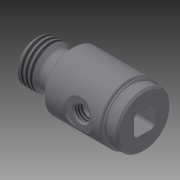
# Autodesk Inventor part: 02R0101_NR_rod_guide
Saved by Autodesk Inventor 2013 (Build 170138000, 138)
## iProperties
Category: PARTsolutions
Company: BIMBA
Created: 2013-01-26
Part Number: 02R0101_NR_rod_guide
Material: Generic
Catalog Web Link: www.cadenas.de
Description: NR Rod Guide-Original Line Cylinders
Vendor: BIMBA
Document SubType Name: Modeling
Designer: actoennies
Manufacturer: BIMBA
Density: 1 g/cm^3
Mass: 3.51503 g
Surface Area: 23.3028 cm^2
Volume: 3.51503 cm^3
PSOL_IDENT_0: {\\10.0.0.242\data_v9\23d-libs\bimba\bimba\bimba_imperial\bimba_full_line\original_line_cylinders\no
PSOL_IDENT_1: n_rotating_air_cylinders\non_rot_rod_guide.prj},201 {VTYP=3D},{NB=02R0101_NR_rod_guide},{LINA=02R010
PSOL_IDENT_2: 1_NR_rod_guide},{NN=NR Rod Guide},{DATE=20.08.2011 07:16:43},{GEOMDATE=16.08.2011 05:39:00},{VERSION
PSOL_IDENT_3: =},{LINEID=30},{LINESUBID=-1},{WBVAR=MNT,DXDE,K,MB}  {NB=02R0101_NR_rod_guide},{LINA=02R0101_NR_rod_
PSOL_IDENT_4: guide},{KT=DUMMY},{PN=02R0101},{BORE=0.56250000},{BOREPN=02},{MNT=},{MNTALG='' , 'Front Nose'},{ACTI
PSOL_IDENT_5: NG=R},{ACTINGALG=R},{DXDE=1},{NR=},{NRALG= '' , 'N/A' },{K=},{T1=},{T2=},{T3=},{T4=},{MB=1},{A1=1.15
PSOL_IDENT_6: 60},{A1N=1.0310},{A1P=1.1560},{A1B=0.0000},{A2=0.3750},{A2N=0.3750},{A2P=0.3750},{A3=0.6250},{A3N=0.
PSOL_IDENT_7: 1250},{A3P=0.6250},{A4=0.1570},{A4N=0.5310},{A4P=0.1570},{A5=0.0250},{A6=0.0000},{A6N=0.2810},{A6P=0
PSOL_IDENT_8: .0000},{A7=0.5000},{A7N=0.6560},{A7P=0.5000},{A8=0.0200},{A8N=0.0200},{A8NR=0.0200},{D1=0.6150},{D1N
PSOL_IDENT_9: =0.6150},{D1P=0.6150},{D1B=0.0000},{D2=0.5725},{D3=0.0000},{D3N=0.4000},{D3P=0.0000},{D4=0.3440},{D4
PSOL_IDENT_10: N=0.2220},{D4P=0.3440},{D4NR=0.3440},{D5=0.1900},{D5N=0.1900},{D5NR=0.1900},{C1=0.030},{C2=0.0200},{
PSOL_IDENT_11: C2N=0.0300},{C2P=0.0200},{C3=0.0100},{C3N=0.0100},{C3P=0.0100},{C4=0.0300},{C4N=0.0300},{C4P=0.0300}
PSOL_IDENT_12: ,{NDM=0.4375},{NDMN=0.4375},{NDMP=0.4375},{TAB=UNF},{D6=0.4355},{D6N=0.4355},{D6P=0.4355},{A9=0.0620
PSOL_IDENT_13: },{A9N=0.0620},{A9P=0.0620},{D7=0.3600},{D7N=0.3600},{D7P=0.3600},{A10=0.0775},{A10N=0.0775},{A10P=0
PSOL_IDENT_14: .0775},{R1=0.0315},{R1N=0.0315},{R1P=0.0315},{D8=0.0000},{D9=0.0000},{D10=0.0000},{A11=0.0000},{A12=
PSOL_IDENT_15: 0.0000},{A13=0.0000},{A14=0.4060},{A14N=0.4060},{A14B=0.0000},{D11=0.0000},{D11N=0.0000},{NDM2=0.190
PSOL_IDENT_16: 0},{NDM2N=0.1900},{NDM2DP=0.0000},{THREAD=0},{HEX=0.2200},{HEXN=0.2200},{S1=0.0000},{B1=0.0000},{B2=
PSOL_IDENT_17: 0.0000},{B22=0.0000},{DB=0.0000},{B3=0.0000},{B4=0.0000},{X1=0.0000},{X2=0.0000},{NDM3=0.0000},{NDM4
PSOL_IDENT_18: =0.0000},{NDM4DP=0.0000},{DD=0.0000},{CB=0.0000},{CBDP=0.0000},{PORT=1},{XT=0.0000},{XT1=0.0000},{XT
PSOL_IDENT_19: 2=0.0000},{NDMH=0.0000},{OD=0.6150},{ID=0.5725},{G=0.0000},{PNUT=0.3750},{TRIM=0},{C11=0.0000},{C22=
PSOL_IDENT_20: 0.0000},{C33=0.0000},{C44=0.0000},{C55=0.0000},{CD1=0.0000},{CD2=0.0000},{CD3=0.0000},{CNDM3=0.0000}
PSOL_IDENT_21: ,{CTAB3=0.0000},{CUSH=0},{XDEDIA=0.19000000},{COR=0.04000000}
CNS_NT: Original Line Cylinders
CNS_NB: 02R0101_NR_rod_guide
CNS_NBSYN: $PN._NR_rod_guide
CNS_LINA: 02R0101_NR_rod_guide
CNS_PN: 02R0101
CNS_BORE: 0.56250000
CNS_BOREPN: 02
CNS_MNT: Front Nose
CNS_MNTALG: '' , 'Front Nose'
CNS_ACTING: R
CNS_ACTINGALG: R
CNS_DXDE: 1
CNS_NRALG: '' , 'N/A'
CNS_K: Standard
CNS_MB: 1
CNS_A1: 1.1560
CNS_A1N: 1.0310
CNS_A1P: 1.1560
CNS_A1B: 0.0000
CNS_A2: 0.3750
CNS_A2N: 0.3750
CNS_A2P: 0.3750
CNS_A3: 0.6250
CNS_A3N: 0.1250
CNS_A3P: 0.6250
CNS_A4: 0.1570
CNS_A4N: 0.5310
CNS_A4P: 0.1570
CNS_A5: 0.0250
CNS_A6: 0.0000
CNS_A6N: 0.2810
CNS_A6P: 0.0000
CNS_A7: 0.5000
CNS_A7N: 0.6560
CNS_A7P: 0.5000
CNS_A8: 0.0200
CNS_A8N: 0.0200
CNS_A8NR: 0.0200
CNS_D1: 0.6150
CNS_D1N: 0.6150
CNS_D1P: 0.6150
CNS_D1B: 0.0000
CNS_D2: 0.5725
CNS_D3: 0.0000
CNS_D3N: 0.4000
CNS_D3P: 0.0000
CNS_D4: 0.3440
CNS_D4N: 0.2220
CNS_D4P: 0.3440
CNS_D4NR: 0.3440
CNS_D5: 0.1900
CNS_D5N: 0.1900
CNS_D5NR: 0.1900
CNS_C1: 0.030
CNS_C2: 0.0200
CNS_C2N: 0.0300
CNS_C2P: 0.0200
CNS_C3: 0.0100
CNS_C3N: 0.0100
CNS_C3P: 0.0100
CNS_C4: 0.0300
CNS_C4N: 0.0300
CNS_C4P: 0.0300
CNS_NDM: 0.4375
CNS_NDMN: 0.4375
CNS_NDMP: 0.4375
CNS_TAB: UNF
CNS_D6: 0.4355
CNS_D6N: 0.4355
CNS_D6P: 0.4355
CNS_A9: 0.0620
CNS_A9N: 0.0620
CNS_A9P: 0.0620
CNS_D7: 0.3600
CNS_D7N: 0.3600
CNS_D7P: 0.3600
CNS_A10: 0.0775
CNS_A10N: 0.0775
CNS_A10P: 0.0775
CNS_R1: 0.0315
CNS_R1N: 0.0315
CNS_R1P: 0.0315
CNS_D8: 0.0000
CNS_D9: 0.0000
CNS_D10: 0.0000
CNS_A11: 0.0000
CNS_A12: 0.0000
CNS_A13: 0.0000
CNS_A14: 0.4060
CNS_A14N: 0.4060
CNS_A14B: 0.0000
CNS_D11: 0.0000
CNS_D11N: 0.0000
CNS_NDM2: 0.1900
CNS_NDM2N: 0.1900
CNS_NDM2DP: 0.0000
CNS_THREAD: 0
CNS_HEX: 0.2200
CNS_HEXN: 0.2200
CNS_S1: 0.0000
CNS_B1: 0.0000
CNS_B2: 0.0000
CNS_B22: 0.0000
CNS_DB: 0.0000
CNS_B3: 0.0000
CNS_B4: 0.0000
CNS_X1: 0.0000
CNS_X2: 0.0000
CNS_NDM3: 0.0000
CNS_NDM4: 0.0000
CNS_NDM4DP: 0.0000
CNS_DD: 0.0000
CNS_CB: 0.0000
CNS_CBDP: 0.0000
CNS_PORT: 1
CNS_XT: 0.0000
CNS_XT1: 0.0000
CNS_XT2: 0.0000
CNS_NDMH: 0.0000
CNS_OD: 0.6150
CNS_ID: 0.5725
CNS_G: 0.0000
CNS_PNUT: 0.3750
CNS_TRIM: 0
CNS_C11: 0.0000
CNS_C22: 0.0000
CNS_C33: 0.0000
CNS_C44: 0.0000
CNS_C55: 0.0000
CNS_CD1: 0.0000
CNS_CD2: 0.0000
CNS_CD3: 0.0000
CNS_CNDM3: 0.0000
CNS_CTAB3: 0.0000
CNS_CUSH: 0.000
CNS_XDEDIA: 0.19000000
CNS_COR: 0.04000000
SUPPLIER: BIMBA
ARTICLENO: 02R0101_NR_rod_guide
BOMINFO: 02R0101_NR_rod_guide
CREATOR: CADENAS GmbH
Title: 02R0101_NR_rod_guide
Author: Cadenas PARTsolutions
Comments: Original Line Cylinders
Autodesk Inventor part; units mm, degrees
sketch "Sketch_2" plane through (0, 0, 0) normal (0, 0, 1) x (1, 0, 0)
  line L0 (9.525, 0) -> (0, 0)
  line L1 (0, 0) -> (0, 4.8006)
  line L2 (0, 4.8006) -> (0.7557, 5.5563)
  line L3 (0.7557, 5.5563) -> (4.6603, 5.5563)
  line L4 (4.6603, 5.5563) -> (5.4159, 4.8006)
  line L5 (5.4159, 4.8006) -> (5.4788, 4.7498)
  arc A0 (5.4788, 4.7498) -> (5.9817, 4.572) centre (5.9817, 5.3721) ccw
  line L6 (5.9817, 4.572) -> (7.1501, 4.572)
  arc A1 (7.1501, 4.572) -> (7.9502, 5.3721) centre (7.1501, 5.3721) ccw
  line L7 (7.9502, 5.3721) -> (7.9502, 5.5309)
  line L8 (7.9502, 5.5309) -> (9.525, 5.5309)
  line L9 (9.525, 5.5309) -> (9.525, 0)
  line L10 (9.525, 0) -> (0, 0)
  constraints: 22 end point, 4 point on circle, 2 centre point
revolve "Revolution1" add sketch "Sketch_2" angle 360 about axis through (9.525, 0, 0) along (1, 0, 0)
thread "Thread1" size "7/16-20 UNF" class "2A" standard "ANSI Unified Screw Threads" full length
sketch "Sketch_3" plane through (0, 0, 0) normal (0, 0, 1) x (1, 0, 0)
  line L0 (29.3624, 0) -> (9.525, 0)
  line L1 (9.525, 0) -> (9.525, 7.0485)
  line L2 (9.525, 7.0485) -> (10.287, 7.8105)
  line L3 (10.287, 7.8105) -> (25.1206, 7.8105)
  line L4 (25.1206, 7.8105) -> (25.3746, 7.5565)
  line L5 (25.3746, 7.5565) -> (25.3746, 6.6357)
  line L6 (25.3746, 6.6357) -> (26.0096, 6.6357)
  line L7 (26.0096, 6.6357) -> (26.6446, 7.2708)
  line L8 (26.6446, 7.2708) -> (28.8544, 7.2708)
  line L9 (28.8544, 7.2708) -> (29.3624, 6.7627)
  line L10 (29.3624, 6.7627) -> (29.3624, 0)
  line L11 (29.3624, 0) -> (9.525, 0)
  constraints: 24 end point
revolve "Revolution2" add sketch "Sketch_3" angle 360 about axis through (29.3624, 0, 0) along (1, 0, 0)
sketch "Sketch_12" plane through (0, 0, 0) normal (0, 1, 0) x (-1, 0, 0)
  line L0 (-19.05, 7.8105) -> (-19.05, -1.016)
  line L1 (-19.05, -1.016) -> (-21.0337, -1.016)
  line L2 (-21.0337, -1.016) -> (-21.0337, 6.3652)
  line L3 (-21.0337, 6.3652) -> (-21.463, 6.7945)
  line L4 (-21.463, 6.7945) -> (-23.0124, 6.7945)
  line L5 (-23.0124, 6.7945) -> (-23.0124, 7.8105)
  line L6 (-23.0124, 7.8105) -> (-19.05, 7.8105)
  line L7 (-19.05, 7.8105) -> (-19.05, -1.016)
  constraints: 16 end point
revolve "Revolution3" cut sketch "Sketch_12" angle 360 about axis through (19.05, 0, 7.8105) along (0, 0, 1)
thread "Thread2" size "10-32 UNF" class "2B" standard "ANSI Unified Screw Threads" length 2.4257 offset 5.3848
sketch "Sketch_47" plane through (0, 0, 0) normal (0, 0, 1) x (1, 0, 0)
  line L0 (26.0096, 0) -> (25.3746, 0)
  line L1 (25.3746, 6.3818) -> (26.0096, 6.3818)
  line L2 (26.0096, 6.3818) -> (26.0096, 6.6357)
  line L3 (26.0096, 6.6357) -> (25.6921, 6.6357)
  line L4 (25.6921, 6.6357) -> (25.4916, 6.8362)
  arc A0 (25.4916, 7.0158) -> (25.4916, 6.8362) centre (25.5814, 6.926) ccw
  line L5 (25.4916, 7.0158) -> (26.2022, 7.7263)
  line L6 (26.2022, 7.7263) -> (26.2022, 7.8105)
  line L7 (26.2022, 7.8105) -> (25.999, 7.8105)
  line L8 (25.999, 7.8105) -> (25.3746, 7.1861)
  line L9 (25.3746, 7.1861) -> (25.3746, 6.3818)
  constraints: 20 end point, 2 point on circle, 1 centre point
revolve "Revolution4" add sketch "Sketch_47" angle 360 about axis through (26.0096, 0, 0) along (1, 0, 0)
sketch "Sketch_33" plane through (0, 0, 0) normal (1, 0, 0) x (0, 1, 0)
  line L0 (1.778, 2.794) -> (-1.778, 2.794)
  arc A0 (-1.778, 2.794) -> (-2.794, 1.778) centre (-1.778, 1.778) ccw
  line L1 (-2.794, 1.778) -> (-2.794, -1.778)
  arc A1 (-2.794, -1.778) -> (-1.778, -2.794) centre (-1.778, -1.778) ccw
  line L2 (-1.778, -2.794) -> (1.778, -2.794)
  arc A2 (1.778, -2.794) -> (2.794, -1.778) centre (1.778, -1.778) ccw
  line L3 (2.794, -1.778) -> (2.794, 1.778)
  arc A3 (2.794, 1.778) -> (1.778, 2.794) centre (1.778, 1.778) ccw
  constraints: 8 end point, 8 point on circle, 4 centre point
extrude "Extrusion1" cut sketch "Sketch_33" along normal blind 58.7248
ref_plane "m1_XY" through (0, 5.5563, 0) normal (0, 0, 1) x (1, 0, 0)
ref_plane "m1_YZ" through (0, 5.5563, 0) normal (1, 0, 0) x (0, 1, 0)
ref_plane "m1_ZX" through (0, 5.5563, 0) normal (0, 1, 0) x (0, 0, 1)
ref_plane "m2_XY" through (0, -5.5563, 0) normal (0, 0, 1) x (1, 0, 0)
ref_plane "m2_YZ" through (0, -5.5563, 0) normal (1, 0, 0) x (0, 1, 0)
ref_plane "m2_ZX" through (0, -5.5563, 0) normal (0, 1, 0) x (0, 0, 1)
ref_plane "s1_XY" through (7.9502, 0, 0) normal (0, 0, 1) x (1, 0, 0)
ref_plane "s1_YZ" through (7.9502, 0, 0) normal (1, 0, 0) x (0, 1, 0)
ref_plane "s1_ZX" through (7.9502, 0, 0) normal (0, 1, 0) x (0, 0, 1)
ref_plane "s2_XY" through (9.525, 0, 0) normal (0, 0, 1) x (1, 0, 0)
ref_plane "s2_YZ" through (9.525, 0, 0) normal (1, 0, 0) x (0, 1, 0)
ref_plane "s2_ZX" through (9.525, 0, 0) normal (0, 1, 0) x (0, 0, 1)
ref_plane "dp1_XY" through (9.525, 5.5309, 0) normal (0, 0, 1) x (1, 0, 0)
ref_plane "dp1_YZ" through (9.525, 5.5309, 0) normal (1, 0, 0) x (0, 1, 0)
ref_plane "dp1_ZX" through (9.525, 5.5309, 0) normal (0, 1, 0) x (0, 0, 1)
ref_plane "dp2_XY" through (9.525, -5.5309, 0) normal (0, 0, 1) x (1, 0, 0)
ref_plane "dp2_YZ" through (9.525, -5.5309, 0) normal (1, 0, 0) x (0, 1, 0)
ref_plane "dp2_ZX" through (9.525, -5.5309, 0) normal (0, 1, 0) x (0, 0, 1)
ref_plane "rod_guide_XY" through (0, 0, 0) normal (1, 0, 0) x (0, 0, -1)
ref_plane "rod_guide_YZ" through (0, 0, 0) normal (0, 0, -1) x (0, 1, 0)
ref_plane "rod_guide_ZX" through (0, 0, 0) normal (0, 1, 0) x (1, 0, 0)
ref_plane "to_tube_XY" through (26.0096, 0, 0) normal (1, 0, 0) x (0, 0, -1)
ref_plane "to_tube_YZ" through (26.0096, 0, 0) normal (0, 0, -1) x (0, 1, 0)
ref_plane "to_tube_ZX" through (26.0096, 0, 0) normal (0, 1, 0) x (1, 0, 0)
ref_plane "to_foot_bracket_XY" through (9.525, 0, 0) normal (1, 0, 0) x (0, 0, -1)
ref_plane "to_foot_bracket_YZ" through (9.525, 0, 0) normal (0, 0, -1) x (0, 1, 0)
ref_plane "to_foot_bracket_ZX" through (9.525, 0, 0) normal (0, 1, 0) x (1, 0, 0)
ref_plane "to_nut_XY" through (9.525, 0, 0) normal (1, 0, 0) x (0, 0, -1)
ref_plane "to_nut_YZ" through (9.525, 0, 0) normal (0, 0, -1) x (0, 1, 0)
ref_plane "to_nut_ZX" through (9.525, 0, 0) normal (0, 1, 0) x (1, 0, 0)
ref_plane "to_trunnion_brackets_XY" through (0, 0, 0) normal (0, 1, 0) x (1, 0, 0)
ref_plane "to_trunnion_brackets_YZ" through (0, 0, 0) normal (1, 0, 0) x (0, 0, -1)
ref_plane "to_trunnion_brackets_ZX" through (0, 0, 0) normal (0, 0, -1) x (0, 1, 0)
ref_plane "to_trunnion_brackets1_XY" through (0, 0, 0) normal (0, 1, 0) x (1, 0, 0)
ref_plane "to_trunnion_brackets1_YZ" through (0, 0, 0) normal (1, 0, 0) x (0, 0, -1)
ref_plane "to_trunnion_brackets1_ZX" through (0, 0, 0) normal (0, 0, -1) x (0, 1, 0)
ref_plane "to_trunnion_brackets2_XY" through (0, 0, 0) normal (0, 1, 0) x (1, 0, 0)
ref_plane "to_trunnion_brackets2_YZ" through (0, 0, 0) normal (1, 0, 0) x (0, 0, -1)
ref_plane "to_trunnion_brackets2_ZX" through (0, 0, 0) normal (0, 0, -1) x (0, 1, 0)
ref_plane "t1_XY" through (9.525, 0, 0) normal (1, 0, 0) x (0, 0, -1)
ref_plane "t1_YZ" through (9.525, 0, 0) normal (0, 0, -1) x (0, 1, 0)
ref_plane "t1_ZX" through (9.525, 0, 0) normal (0, 1, 0) x (1, 0, 0)
ref_plane "port_XY" through (19.05, 0, 0) normal (0, 0, 1) x (1, 0, 0)
ref_plane "port_YZ" through (19.05, 0, 0) normal (1, 0, 0) x (0, 1, 0)
ref_plane "port_ZX" through (19.05, 0, 0) normal (0, 1, 0) x (0, 0, 1)
ref_plane "rod_guide_1_XY" through (0, 0, 0) normal (1, 0, 0) x (0, 0, -1)
ref_plane "rod_guide_1_YZ" through (0, 0, 0) normal (0, 0, -1) x (0, 1, 0)
ref_plane "rod_guide_1_ZX" through (0, 0, 0) normal (0, 1, 0) x (1, 0, 0)
ref_plane "rod_guide_11_XY" through (0, 0, 0) normal (1, 0, 0) x (0, 0, -1)
ref_plane "rod_guide_11_YZ" through (0, 0, 0) normal (0, 0, -1) x (0, 1, 0)
ref_plane "rod_guide_11_ZX" through (0, 0, 0) normal (0, 1, 0) x (1, 0, 0)
body "Solid1"
